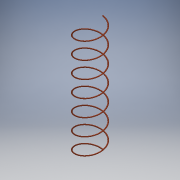
# Autodesk Inventor part: Ground_Antenna700mm_Helix
Saved by Autodesk Inventor 2018 (Build 220112000, 112)
## iProperties
Created: 2018-09-26
Part Number: Ground_Antenna700mm_Helix
Material: Copper
Document SubType Name: Modeling
Designer: Bradley
Density: 8.94 g/cm^3
Appearance: Copper - Satin
Mass: 1079.53 g
Surface Area: 3002.58 cm^2
Volume: 120.753 cm^3
Author: Bradley
Autodesk Inventor part; units mm, degrees
ref_plane "YZ Plane" through (0, 0, 0) normal (1, 0, 0) x (0, 1, 0)
ref_plane "XZ Plane" through (0, 0, 0) normal (0, 1, 0) x (-1, 0, 0)
ref_plane "XY Plane" through (0, 0, 0) normal (0, 0, 1) x (1, 0, 0)
sketch "Sketch1" plane through (0, 0, 0) normal (1, 0, 0) x (0, 1, 0)
  circle A0 centre (123.4125, 0) radius 4.7625
  circle A1 centre (123.4125, 0) radius 3.9497
  line L0 (0, 0) -> (118.65, 0) construction
  line L1 (0, 0) -> (0, 158.6)
  dimension "d0" = 9.525
  dimension "d1" = 7.8994
  dimension "d2" = 237.3
  dimension "d3" = 158.6
  constraints: 4 end point, 1 centre point, 1 coincident, 1 horizontal, 1 horizontal alignment, 1 point on line, 1 vertical, 2 other
  measures "d1" diameter of A1
  measures "d2" diameter of L0.end L1
  measures "d3" distance of L0.start L1.end
coil "Coil1" sketch "Sketch1" operation add axis through (0, 0, 0) along (0, 0, 1) pitch 158.6 turns 7 hand right
equation "\"d4\" = d3"
body "Solid1"
